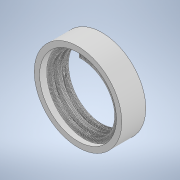
# Autodesk Inventor part: vial thread insert
Saved by Autodesk Inventor 2022 (Build 260153000, 153)
## iProperties
Created: 2022-06-21
Part Number: vial thread insert
Material: Generic
Document SubType Name: Modeling
Designer: efred
Density: 1 g/cm^3
Appearance: Default
Author: efred
Autodesk Inventor part; units mm, degrees
ref_plane "YZ Plane" through (0, 0, 0) normal (1, 0, 0) x (0, 1, 0)
ref_plane "XZ Plane" through (0, 0, 0) normal (0, 1, 0) x (-1, 0, 0)
ref_plane "XY Plane" through (0, 0, 0) normal (0, 0, 1) x (1, 0, 0)
sketch "Sketch1" plane through (-9.8257, 10.5269, -8.5) normal (0, 0, -1) x (-1, 0, 0)
  circle A0 centre (-9.826, -10.5267) radius 14.4003 projected
  circle A1 centre (-9.826, -10.5267) radius 16.4003
  point P0 (-9.8257, -10.5269)
  dimension "d0" = 2
  constraints: 1 centre point
  measures "d0" radial gap between concentric circles of A0 A1
extrude "Extrusion1" add sketch "Sketch1" against normal blind 9
body "Solid1"
